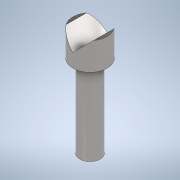
# Autodesk Inventor part: Yunque V
Saved by Autodesk Inventor 2020 (Build 240168000, 168)
## iProperties
Created: 2020-09-17
Part Number: Yunque V
Material: Steel AISI 1045 HV HR
Document SubType Name: Modeling
Designer: aaron
Density: 7.85 g/cm^3
Appearance: Steel - Polished
Author: aaron
Autodesk Inventor part; units mm, degrees
ref_plane "YZ Plane" through (0, 0, 0) normal (1, 0, 0) x (0, 1, 0)
ref_plane "XZ Plane" through (0, 0, 0) normal (0, 1, 0) x (-1, 0, 0)
ref_plane "XY Plane" through (0, 0, 0) normal (0, 0, 1) x (1, 0, 0)
sketch "Sketch1" plane through (0, 0, 0) normal (0, 0, 1) x (1, 0, 0)
  line L0 (-4.7371, 12.7) -> (3.2004, 12.7)
  line L1 (3.2004, 12.7) -> (3.2004, 0)
  line L2 (3.2004, 0) -> (0, 0)
  line L3 (0, 0) -> (0, -38.1)
  line L4 (0, -38.1) -> (-4.7371, -38.1)
  line L5 (-4.7371, -38.1) -> (-4.7371, 12.7)
  dimension "d0" = 9.4742
  dimension "d1" = 12.7
  dimension "d2" = 15.875
  dimension "d3" = 50.8
  constraints: 12 end point, 5 perpendicular, 1 coincident, 1 horizontal
  measures "d0" diameter of L3 L5
  measures "d1" distance between parallel lines of L2 L0
  measures "d2" diameter of L1 L5
  measures "d3" distance between parallel lines of L4 L0
revolve "Revolution1" add sketch "Sketch1" angle 360 about axis through (-4.7371, -38.1, 0) along (0, 1, 0)
sketch "Sketch3" plane through (0, 0, 0) normal (0, 0, 1) x (1, 0, 0)
  line L0 (-12.6746, 12.7) -> (3.2004, 12.7) projected
  line L1 (-12.6746, 0) -> (3.2004, 0) projected
  line L2 (-12.6746, 12.7) -> (3.2004, 12.7) projected
  line L3 (-11.0871, 12.7) -> (-4.7371, 6.35)
  line L4 (-4.7371, 6.35) -> (1.6129, 12.7)
  line L5 (-12.6746, 12.7) -> (3.2004, 12.7) projected
  line L6 (3.2004, 12.7) -> (3.2004, 0) projected
  line L7 (3.2004, 0) -> (0, 0) projected
  line L8 (0, 0) -> (0, -38.1) projected
  line L9 (0, -38.1) -> (-9.4742, -38.1) projected
  line L10 (-9.4742, -38.1) -> (-9.4742, 0) projected
  line L11 (-9.4742, 0) -> (-12.6746, 0) projected
  line L12 (-12.6746, 0) -> (-12.6746, 12.7) projected
  dimension "d5" = 1.5875
  dimension "d6" = 1.5875
  dimension "d7" = 45
  dimension "d8" = 45
  constraints: 4 end point, 2 point on line
  measures "d5" distance from line of L12 L3.start
  measures "d6" distance from line of L6 L4.end
  measures "d7" angle of L0 L3
  measures "d8" angle of L0 L4
extrude "Extrusion1" cut sketch "Sketch3" along normal mid plane 25.4 contours L0 L4 L3
body "Solid1"
